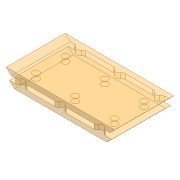
# Autodesk Inventor part: flange7-42mm
Saved by Autodesk Inventor 2021 (Build 250183000, 183)
## iProperties
Created: 2022-10-18
Part Number: flange7-42mm
Material: Rubber, Silicone
Document SubType Name: Modeling
Designer: alyn649
Density: 1.25 g/cm^3
Appearance: Clear - Yellow(1)
Author: alyn649
Autodesk Inventor part; units mm, degrees
ref_plane "YZ Plane" through (0, 0, 0) normal (1, 0, 0) x (0, 1, 0)
ref_plane "XZ Plane" through (0, 0, 0) normal (0, 1, 0) x (-1, 0, 0)
ref_plane "XY Plane" through (0, 0, 0) normal (0, 0, 1) x (1, 0, 0)
sketch "Sketch2" plane through (0, 0, 0) normal (0, 0, 1) x (1, 0, 0)
  line L0 (-15.68, 0) -> (15.68, 0)
  line L1 (15.68, 0) -> (14.1267, -1.5)
  line L2 (14.1267, -1.5) -> (-14.1267, -1.5)
  line L3 (-14.1267, -1.5) -> (-15.68, 0)
  line L4 (-8.8153, 7.7377) -> (-16.0231, 7.7377) construction
  line L5 (15.68, 0) -> (19.7494, 0) construction
  point P0 (0, 0)
  point P1 (0, 0)
  dimension "d0" = 31.36
  dimension "d1" = 136
  dimension "d2" = 136
  dimension "d3" = 1.5
  constraints: 12 end point, 3 horizontal, 1 coincident, 1 midpoint, 1 parallel
  measures "d0" distance of L0.start L0.end
  measures "d1" angle of L3 L4
  measures "d2" angle of L5 L1
  measures "d3" distance between parallel lines of L0 L2
extrude "Extrusion1" add sketch "Sketch2" along normal mid plane 18
sketch "Sketch3" plane through (-15.68, 0, 9) normal (0, 1, 0) x (1, 0, 0)
  circle A0 centre (3.68, 13.5) radius 1
  line L0 (0, 18) -> (31.36, 18) construction
  circle A1 centre (3.68, 18) radius 1 construction
  arc A2 (2.814, 17.5) -> (1.9479, 18) centre (1.9479, 17) ccw
  arc A3 (2.814, 17.5) -> (4.546, 17.5) centre (3.68, 18) ccw
  arc A4 (5.4121, 18) -> (4.546, 17.5) centre (5.4121, 17) ccw
  line L1 (1.9479, 18) -> (8.6251, 18)
  point P0 (15.68, 9)
  point P1 (5.4121, 18)
  dimension "d6" = 12
  dimension "d7" = 4.5
  dimension "d8" = 2
  dimension "d9" = 2
  dimension "d10" = 1
  dimension "d11" = 1
  constraints: 8 point on circle, 7 tangent, 5 centre point, 4 point on line, 2 end point, 1 vertical alignment
  measures "d6" horizontal distance of A0.centre point (15.68, 9)
  measures "d7" vertical distance of A0.centre point (15.68, 9)
  measures "d8" diameter of A1
  measures "d9" diameter of A0
  measures "d10" radius of A2
  measures "d11" radius of A4
extrude "Extrusion2" add sketch "Sketch3" along normal blind 1.5
mirror "Mirror6" about plane through (0, 0, 0) normal (0, 0, 1) of "Extrusion2"
pattern_linear "Rectangular Pattern1" count 3 spacing 12 along (1, 0, 0) of "Extrusion2", "Mirror6"
sketch "Sketch6" plane through (0, 0, 9) normal (0, 0, 1) x (1, 0, 0)
  line L0 (-14.1267, -1.5) -> (14.1267, -1.5) construction
  line L1 (14.1267, -1.5) -> (15.68, 0) construction
  line L2 (15.68, 0) -> (13.7321, 0) construction
  line L3 (13.7321, 0) -> (13.7321, 1.5) construction
  line L4 (13.7321, 1.5) -> (10.2679, 1.5) construction
  line L5 (10.2679, 0) -> (10.2679, 1.5) construction
  line L6 (10.2679, 0) -> (1.7321, 0) construction
  line L7 (1.7321, 0) -> (1.7321, 1.5) construction
  line L8 (1.7321, 1.5) -> (-1.7321, 1.5) construction
  line L9 (-1.7321, 0) -> (-1.7321, 1.5) construction
  line L10 (-1.7321, 0) -> (-10.2679, 0) construction
  line L11 (-10.2679, 0) -> (-10.2679, 1.5) construction
  line L12 (-10.2679, 1.5) -> (-13.7321, 1.5) construction
  line L13 (-13.7321, 0) -> (-13.7321, 1.5) construction
  line L14 (-13.7321, 0) -> (-15.68, 0) construction
  line L15 (-15.68, 0) -> (-14.1267, -1.5) construction
  line L16 (-16.6273, 3) -> (-15.074, 1.5)
  line L17 (-15.074, 1.5) -> (15.074, 1.5)
  line L18 (15.074, 1.5) -> (16.6273, 3)
  line L19 (-16.6273, 3) -> (16.6273, 3)
  point P0 (0, 0)
  point P1 (0, 1.5)
  dimension "d26" = 1.5
  dimension "d27" = 1.5
  dimension "d28" = 1.5
  constraints: 8 end point, 2 horizontal, 2 midpoint, 2 parallel
  measures "d26" distance between parallel lines of L16 L15
  measures "d27" distance between parallel lines of L18 L1
  measures "d28" distance between parallel lines of L19 L17
extrude "Extrusion5" add sketch "Sketch6" against normal blind 18
equation "\"d2\" = d1"
equation "\"d11\" = d10"
body "Solid1"
